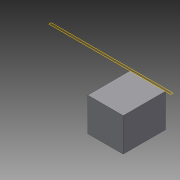
# Autodesk Inventor part: supporto_manicotto_Z
Saved by Autodesk Inventor 2014 SP1 (Build 180222100, 222)
## iProperties
Created: 2015-04-08
Part Number: supporto_manicotto_Z
Material: Generic
Document SubType Name: Modeling
Designer: Giorgio Nuzzo
Density: 1 g/cm^3
Appearance: Default
d0: 32,000 mm
d1: 30,000 mm
d2: 0,00 deg
Author: Giorgio Nuzzo
Autodesk Inventor part; units mm, degrees
ref_plane "YZ Plane" through (0, 0, 0) normal (1, 0, 0) x (0, 1, 0)
ref_plane "XZ Plane" through (0, 0, 0) normal (0, 1, 0) x (-1, 0, 0)
ref_plane "XY Plane" through (0, 0, 0) normal (0, 0, 1) x (1, 0, 0)
ref_plane "Work Plane1" through (99.21, -213.5, 317.498) normal (0, 0, 1) x (-1, 0, 0)
sketch "Sketch1" plane through (99.21, -213.5, 317.498) normal (0, 0, 1) x (-1, 0, 0)
  line L0 (99.8999, 40) -> (0, 40) construction
  circle A0 centre (15.057, 25.15) radius 5 construction
  line L1 (44.96, 36) -> (42.96, 36) construction
  line L2 (42.96, 36) -> (42.96, 37) construction
  line L3 (42.96, 37) -> (40.96, 37) construction
  line L4 (40.96, 37) -> (40.96, 38) construction
  line L5 (40.96, 38) -> (39.71, 38) construction
  arc A1 (39.71, 38) -> (37.21, 35.5) centre (39.71, 35.5) ccw construction
  line L6 (37.21, 35.5) -> (37.21, 34.25) construction
  line L7 (37.21, 34.25) -> (38.21, 34.25) construction
  line L8 (38.21, 34.25) -> (38.21, 32.25) construction
  line L9 (38.21, 32.25) -> (39.21, 32.25) construction
  line L10 (39.21, 32.25) -> (39.21, 30.25) construction
  line L11 (39.21, 30.25) -> (44.96, 30.25) construction
  line L12 (44.96, 30.25) -> (44.96, 36) construction
  line L13 (39.21, 20.25) -> (39.21, 18.25) construction
  line L14 (39.21, 18.25) -> (38.21, 18.25) construction
  line L15 (38.21, 18.25) -> (38.21, 16.25) construction
  line L16 (38.21, 16.25) -> (37.21, 16.25) construction
  line L17 (37.21, 16.25) -> (37.21, 15) construction
  arc A2 (37.21, 15) -> (39.71, 12.5) centre (39.71, 15) ccw construction
  line L18 (39.71, 12.5) -> (40.96, 12.5) construction
  line L19 (40.96, 12.5) -> (40.96, 13.5) construction
  line L20 (40.96, 13.5) -> (42.96, 13.5) construction
  line L21 (42.96, 13.5) -> (42.96, 14.5) construction
  line L22 (42.96, 14.5) -> (44.96, 14.5) construction
  line L23 (44.96, 14.5) -> (44.96, 20.25) construction
  line L24 (44.96, 20.25) -> (39.21, 20.25) construction
  line L25 (54.96, 14.5) -> (56.96, 14.5) construction
  line L26 (56.96, 14.5) -> (56.96, 13.5) construction
  line L27 (56.96, 13.5) -> (58.96, 13.5) construction
  line L28 (58.96, 13.5) -> (58.96, 12.5) construction
  line L29 (58.96, 12.5) -> (60.21, 12.5) construction
  arc A3 (60.21, 12.5) -> (62.71, 15) centre (60.21, 15) ccw construction
  line L30 (62.71, 15) -> (62.71, 16.25) construction
  line L31 (62.71, 16.25) -> (61.71, 16.25) construction
  line L32 (61.71, 16.25) -> (61.71, 18.25) construction
  line L33 (61.71, 18.25) -> (60.71, 18.25) construction
  line L34 (60.71, 18.25) -> (60.71, 20.25) construction
  line L35 (60.71, 20.25) -> (54.96, 20.25) construction
  line L36 (54.96, 20.25) -> (54.96, 14.5) construction
  line L37 (60.71, 30.25) -> (60.71, 32.25) construction
  line L38 (60.71, 32.25) -> (61.71, 32.25) construction
  line L39 (61.71, 32.25) -> (61.71, 34.25) construction
  line L40 (61.71, 34.25) -> (62.71, 34.25) construction
  line L41 (62.71, 34.25) -> (62.71, 35.5) construction
  arc A4 (62.71, 35.5) -> (60.21, 38) centre (60.21, 35.5) ccw construction
  line L42 (60.21, 38) -> (58.96, 38) construction
  line L43 (58.96, 38) -> (58.96, 37) construction
  line L44 (58.96, 37) -> (56.96, 37) construction
  line L45 (56.96, 37) -> (56.96, 36) construction
  line L46 (56.96, 36) -> (54.96, 36) construction
  line L47 (54.96, 36) -> (54.96, 30.25) construction
  line L48 (54.96, 30.25) -> (60.71, 30.25) construction
  line L49 (53.142, 27.7249) -> (52.4349, 28.432) construction
  line L50 (52.4349, 28.432) -> (51.3385, 27.3356) construction
  arc A5 (51.3385, 27.3356) -> (48.5815, 27.3356) centre (49.96, 25.25) ccw construction
  line L51 (48.5815, 27.3356) -> (47.4852, 28.432) construction
  line L52 (47.4852, 28.432) -> (46.7781, 27.7249) construction
  line L53 (46.7781, 27.7249) -> (47.8744, 26.6285) construction
  arc A6 (47.8744, 26.6285) -> (47.8744, 23.8715) centre (49.96, 25.25) ccw construction
  line L54 (47.8744, 23.8715) -> (46.7781, 22.7751) construction
  line L55 (46.7781, 22.7751) -> (47.4852, 22.068) construction
  line L56 (47.4852, 22.068) -> (48.5815, 23.1644) construction
  arc A7 (48.5815, 23.1644) -> (51.3385, 23.1644) centre (49.96, 25.25) ccw construction
  line L57 (51.3385, 23.1644) -> (52.4349, 22.068) construction
  line L58 (52.4349, 22.068) -> (53.142, 22.7751) construction
  line L59 (53.142, 22.7751) -> (52.0456, 23.8715) construction
  arc A8 (52.0456, 23.8715) -> (52.0456, 26.6285) centre (49.96, 25.25) ccw construction
  line L60 (52.0456, 26.6285) -> (53.142, 27.7249) construction
  line L61 (60.21, 27.75) -> (60.21, 29.25) construction
  line L62 (60.21, 29.25) -> (54.96, 29.25) construction
  line L63 (54.96, 29.25) -> (54.96, 21.25) construction
  line L64 (54.96, 21.25) -> (60.21, 21.25) construction
  line L65 (60.21, 21.25) -> (60.21, 22.75) construction
  line L66 (60.21, 22.75) -> (61.71, 22.75) construction
  line L67 (61.71, 22.75) -> (61.71, 19.25) construction
  line L68 (61.71, 19.25) -> (62.71, 19.25) construction
  line L69 (62.71, 19.25) -> (62.71, 17.25) construction
  line L70 (62.71, 17.25) -> (63.71, 17.25) construction
  line L71 (63.71, 17.25) -> (63.71, 15) construction
  arc A9 (60.21, 11.5) -> (63.71, 15) centre (60.21, 15) ccw construction
  line L72 (60.21, 11.5) -> (57.96, 11.5) construction
  line L73 (57.96, 11.5) -> (57.96, 12.5) construction
  line L74 (57.96, 12.5) -> (55.96, 12.5) construction
  line L75 (55.96, 12.5) -> (55.96, 13.5) construction
  line L76 (55.96, 13.5) -> (52.46, 13.5) construction
  line L77 (52.46, 13.5) -> (52.46, 15) construction
  line L78 (52.46, 15) -> (53.96, 15) construction
  line L79 (53.96, 15) -> (53.96, 20.25) construction
  line L80 (53.96, 20.25) -> (45.96, 20.25) construction
  line L81 (45.96, 20.25) -> (45.96, 15) construction
  line L82 (45.96, 15) -> (47.46, 15) construction
  line L83 (47.46, 15) -> (47.46, 13.5) construction
  line L84 (47.46, 13.5) -> (43.96, 13.5) construction
  line L85 (43.96, 13.5) -> (43.96, 12.5) construction
  line L86 (43.96, 12.5) -> (41.96, 12.5) construction
  line L87 (41.96, 12.5) -> (41.96, 11.5) construction
  line L88 (41.96, 11.5) -> (39.71, 11.5) construction
  arc A10 (36.21, 15) -> (39.71, 11.5) centre (39.71, 15) ccw construction
  line L89 (36.21, 15) -> (36.21, 17.25) construction
  line L90 (36.21, 17.25) -> (37.21, 17.25) construction
  line L91 (37.21, 17.25) -> (37.21, 19.25) construction
  line L92 (37.21, 19.25) -> (38.21, 19.25) construction
  line L93 (38.21, 19.25) -> (38.21, 22.75) construction
  line L94 (38.21, 22.75) -> (39.71, 22.75) construction
  line L95 (39.71, 22.75) -> (39.71, 21.25) construction
  line L96 (39.71, 21.25) -> (44.96, 21.25) construction
  line L97 (44.96, 21.25) -> (44.96, 29.25) construction
  line L98 (44.96, 29.25) -> (39.71, 29.25) construction
  line L99 (39.71, 29.25) -> (39.71, 27.75) construction
  line L100 (39.71, 27.75) -> (38.21, 27.75) construction
  line L101 (38.21, 27.75) -> (38.21, 31.25) construction
  line L102 (38.21, 31.25) -> (37.21, 31.25) construction
  line L103 (37.21, 31.25) -> (37.21, 33.25) construction
  line L104 (37.21, 33.25) -> (36.21, 33.25) construction
  line L105 (36.21, 33.25) -> (36.21, 35.5) construction
  arc A11 (39.71, 39) -> (36.21, 35.5) centre (39.71, 35.5) ccw construction
  line L106 (39.71, 39) -> (41.96, 39) construction
  line L107 (41.96, 39) -> (41.96, 38) construction
  line L108 (41.96, 38) -> (43.96, 38) construction
  line L109 (43.96, 38) -> (43.96, 37) construction
  line L110 (43.96, 37) -> (47.46, 37) construction
  line L111 (47.46, 37) -> (47.46, 35.5) construction
  line L112 (47.46, 35.5) -> (45.96, 35.5) construction
  line L113 (45.96, 35.5) -> (45.96, 30.25) construction
  line L114 (45.96, 30.25) -> (53.96, 30.25) construction
  line L115 (53.96, 30.25) -> (53.96, 35.5) construction
  line L116 (53.96, 35.5) -> (52.46, 35.5) construction
  line L117 (52.46, 35.5) -> (52.46, 37) construction
  line L118 (52.46, 37) -> (55.96, 37) construction
  line L119 (55.96, 37) -> (55.96, 38) construction
  line L120 (55.96, 38) -> (57.96, 38) construction
  line L121 (57.96, 38) -> (57.96, 39) construction
  line L122 (57.96, 39) -> (60.21, 39) construction
  arc A12 (63.71, 35.5) -> (60.21, 39) centre (60.21, 35.5) ccw construction
  line L123 (63.71, 35.5) -> (63.71, 33.25) construction
  line L124 (63.71, 33.25) -> (62.71, 33.25) construction
  line L125 (62.71, 33.25) -> (62.71, 31.25) construction
  line L126 (62.71, 31.25) -> (61.71, 31.25) construction
  line L127 (61.71, 31.25) -> (61.71, 27.75) construction
  line L128 (61.71, 27.75) -> (60.21, 27.75) construction
  line L129 (0, 0) -> (0, 2) construction
  line L130 (0, 2) -> (99.8999, 2) construction
  line L131 (99.8999, 0) -> (99.8999, 2) construction
  line L132 (99.8999, 0) -> (0, 0) construction
  line L133 (99.8999, 42) -> (99.8999, 40) construction
  line L134 (99.8999, 40) -> (0, 40) construction
  line L135 (0, 42) -> (0, 40) construction
  line L136 (0, 42) -> (99.8999, 42) construction
  line L137 (0, 40) -> (32, 40)
  line L138 (32, 40) -> (32, 2)
  line L139 (32, 2) -> (0, 2)
  line L140 (0, 2) -> (0, 40)
  point P0 (99.21, -213.5)
  dimension "d0" = 32
  constraints: 280 end point, 63 horizontal, 62 vertical, 24 point on circle, 13 centre point, 2 parallel, 1 perpendicular, 1 point on line, 184 other
  measures "d0" distance between parallel lines of L140 L138
extrude "Extrusion1" add sketch "Sketch1" against normal blind 30
body "Solid1"
